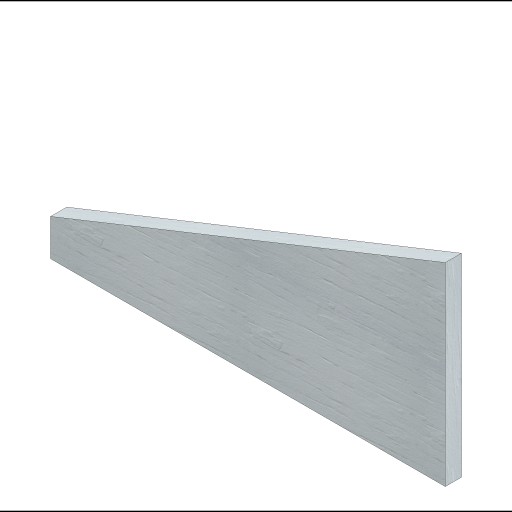
# Autodesk Inventor part: Inlet Support Leg Proto 1
Saved by Autodesk Inventor 2023 (Build 270158000, 158)
## iProperties
Created: 2023-01-19
Part Number: Inlet Support Leg Proto 1
Material: Wood (Oak)
Document SubType Name: Modeling
Designer: kamer
Density: 0.76 g/cm^3
Appearance: Wood - Painted White
Author: kamer
Autodesk Inventor part; units mm, degrees
ref_plane "YZ Plane" through (0, 0, 0) normal (1, 0, 0) x (0, 1, 0)
ref_plane "XZ Plane" through (0, 0, 0) normal (0, 1, 0) x (-1, 0, 0)
ref_plane "XY Plane" through (0, 0, 0) normal (0, 0, 1) x (1, 0, 0)
sketch "Sketch2" plane through (0, 0, 0) normal (0, 0, 1) x (1, 0, 0)
  line L0 (0, 0) -> (38.1, 0)
  line L1 (38.1, 0) -> (38.1, 11.938) construction
  line L2 (38.1, 11.938) -> (0, 11.938)
  line L3 (0, 11.938) -> (0, 0)
  line L4 (0, 11.938) -> (330.3077, 143.6506)
  line L5 (0, 11.938) -> (355.6, 11.938) construction
  line L6 (38.1, 0) -> (38.1, 27.1307)
  line L7 (330.3077, 143.6506) -> (330.3077, 0)
  line L8 (330.3077, 0) -> (38.1, 0)
  dimension "d5" = 11.938
  dimension "d6" = 38.1
  dimension "d7" = 355.6
  dimension "d8" = 21.74
  constraints: 18 end point, 3 perpendicular, 2 horizontal, 2 parallel, 1 equal length, 1 point on line, 1 vertical
  measures "d5" distance of L2.end L0.start
  measures "d6" distance of L1.end L2.end
  measures "d7" distance of L2.end L4.end
  measures "d8" angle of L5 L4
extrude "Extrusion1" add sketch "Sketch2" along normal blind 11.938 contours L6 L4 L7 L8
body "Solid1"
